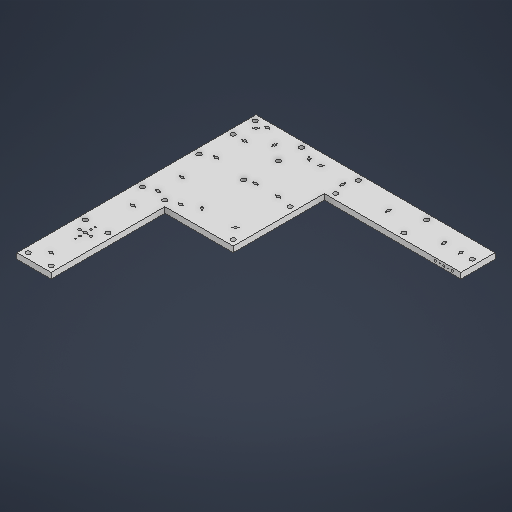
# Autodesk Inventor part: Baseplate Illum V3 L
Saved by Autodesk Inventor 2026 (Build 300175000, 175)
## iProperties
Created: 2026-02-09
Part Number: Baseplate Illum V3 L
Material: Generic
Document SubType Name: Modeling
Designer: FiolkaLab
Density: 1 g/cm^3
Appearance: Default
Author: FiolkaLab
Autodesk Inventor part; units mm, degrees
ref_plane "YZ Plane" through (0, 0, 0) normal (1, 0, 0) x (0, 1, 0)
ref_plane "XZ Plane" through (0, 0, 0) normal (0, 1, 0) x (-1, 0, 0)
ref_plane "XY Plane" through (0, 0, 0) normal (0, 0, 1) x (1, 0, 0)
sketch "Sketch1" plane through (0, 0, 0) normal (0, 1, 0) x (-1, 0, 0)
  line L0 (38.1, 0) -> (-38.1, 0)
  line L1 (-38.1, 0) -> (-38.1, 457.2)
  line L2 (-38.1, 457.2) -> (38.1, 457.2)
  line L3 (38.1, 457.2) -> (38.1, 0)
  point P0 (0, 0)
  dimension "d0" = 76.2
  dimension "d1" = 38.1
  dimension "d2" = 457.2
  constraints: 8 end point, 2 parallel, 1 horizontal, 1 perpendicular
  measures "d0" distance of L1.end L2.end
  measures "d1" distance of L0.start point (0, 0)
  measures "d2" distance of L2.end L0.start
extrude "Extrusion1" add sketch "Sketch1" along normal blind 12.7
sketch "Sketch2" plane through (0, 0, 0) normal (0, -1, 0) x (1, 0, 0)
  line L0 (38.1, 457.2) -> (38.1, 0) projected
  line L1 (-38.1, 457.2) -> (38.1, 457.2) projected
  point P0 (0, 0)
  point P1 (0, 419.1)
  dimension "d12" = 38.1
  dimension "d13" = 38.1
  measures "d12" distance from line of L0 point (0, 419.1)
  measures "d13" distance from line of L1 point (0, 419.1)
hole "Hole1" at (0, 0, 419.1) direction (0, 1, 0) diameter 6.35 end through all counterbore diameter 10.16 counterbore depth 7.62
sketch "Sketch3" plane through (0, 12.7, 0) normal (0, 1, 0) x (1, 0, 0)
  circle A0 centre (-5.004, -419.1) radius 1.0125
  circle A1 centre (5.004, -419.1) radius 1.0125
  circle A2 centre (0, -419.1) radius 3.175 projected
  point P0 (0, 0)
  dimension "d14" = 2.025
  dimension "d15" = 2.025
  dimension "d16" = 5.004
  dimension "d17" = 5.004
  constraints: 2 centre point
  measures "d14" diameter of A0
  measures "d15" diameter of A1
  measures "d16" distance of A2.centre A0.centre
  measures "d17" distance of A2.centre A1.centre
extrude "Extrusion2" cut sketch "Sketch3" against normal blind 4.445 contours A0 | A1
pattern_linear "Rectangular Pattern1" count 2 spacing 76.744 along (0, 0, -1) of "Hole1", "Extrusion2"
pattern_linear "Rectangular Pattern2" count 2 spacing 182.468 along (0, 0, -1) of "Hole1", "Extrusion2"
pattern_linear "Rectangular Pattern3" count 2 spacing 238.5038 along (0, 0, -1) of "Hole1", "Extrusion2"
sketch "Sketch5" plane through (0, 12.7, 0) normal (0, 1, 0) x (1, 0, 0)
  line L0 (38.1, 0) -> (-38.1, 0) projected
  line L1 (-38.1, 0) -> (495.3, 0)
  line L2 (495.3, 0) -> (495.3, 76.2)
  line L3 (495.3, 76.2) -> (-38.1, 76.2)
  line L4 (-38.1, 76.2) -> (-38.1, 0)
  point P0 (0, 0)
  point P1 (38.1, 0)
  dimension "d31" = 76.2
  dimension "d32" = 533.4
  constraints: 8 end point, 2 parallel, 1 horizontal, 1 perpendicular
  measures "d31" distance of L3.end L0.end
  measures "d32" distance of L2.end L3.end
extrude "Extrusion3" add sketch "Sketch5" against normal blind 12.7
sketch "Sketch6" plane through (0, 0, 0) normal (0, -1, 0) x (1, 0, 0)
  line L0 (-38.1, 457.2) -> (-38.1, -76.2) projected
  line L1 (-38.1, -76.2) -> (495.3, -76.2) projected
  point P0 (0, 0)
  point P1 (-12.0376, -50.1336)
  dimension "d42" = 26.0624
  dimension "d43" = 26.0664
  measures "d42" distance from line of L0 point (-12.038, -50.134)
  measures "d43" distance from line of L1 point (-12.038, -50.134)
hole "Hole2" at (-12.0376, 0, -50.1336) direction (0, 1, 0) diameter 6.35 end through all counterbore diameter 10.16 counterbore depth 7.62
sketch "Sketch11" plane through (0, 12.7, 0) normal (0, 1, 0) x (1, 0, 0)
  circle A0 centre (-17.0416, 46.9586) radius 1.0125
  circle A1 centre (-7.0336, 53.3086) radius 1.0125
  circle A2 centre (-12.0376, 50.1336) radius 3.175 projected
  circle A3 centre (-15.576, 46.5952) radius 1.0125
  circle A4 centre (-8.4992, 53.672) radius 1.0125
  point P0 (0, 0)
  dimension "d67" = 2.025
  dimension "d68" = 2.025
  dimension "d69" = 5.004
  dimension "d70" = 3.175
  dimension "d71" = 5.004
  dimension "d72" = 3.175
  dimension "d404" = 2.025
  dimension "d405" = 2.025
  dimension "d406" = 5.004
  dimension "d407" = 5.004
  constraints: 4 centre point
  measures "d67" diameter of A0
  measures "d68" diameter of A1
  measures "d69" horizontal distance of A2.centre A0.centre
  measures "d70" vertical distance of A2.centre A0.centre
  measures "d71" horizontal distance of A2.centre A1.centre
  measures "d72" vertical distance of A2.centre A1.centre
  measures "d404" diameter of A3
  measures "d405" diameter of A4
  measures "d406" distance of A2.centre A3.centre
  measures "d407" distance of A2.centre A4.centre
extrude "Extrusion6" [suppressed]
sketch "Sketch12" plane through (38.1, 0, 457.2) normal (1, 0, 0) x (0, 0, -1)
  line L0 (457.2, 0) -> (457.2, 12.7) projected
  line L1 (0, 0) -> (457.2, 0) projected
  line L2 (457.2, 12.7) -> (254, 12.7)
  line L3 (254, 12.7) -> (254, 0)
  line L4 (254, 0) -> (457.2, 0)
  line L5 (457.2, 0) -> (457.2, 12.7)
  dimension "d77" = 203.2
  constraints: 8 end point, 2 parallel, 1 horizontal, 1 perpendicular, 1 point on line
  measures "d77" distance of L4.end L3.end
extrude "Extrusion7" add sketch "Sketch12" along normal blind 152.4
sketch "Sketch13" plane through (0, 0, 0) normal (0, -1, 0) x (1, 0, 0)
  circle A0 centre (0, 180.5962) radius 5.08 projected
  line L0 (38.1, 203.2) -> (190.5, 203.2) projected
  point P0 (0, 0)
  point P1 (50.8, 180.7682)
  dimension "d87" = 50.8
  dimension "d318" = 0.172
  measures "d87" horizontal distance of A0.centre point (50.8, 180.768)
  measures "d318" vertical distance of point (50.8, 180.768) A0.centre
hole "Hole4" at (50.8, 0, 180.7682) direction (0, 1, 0) diameter 6.35 end through all counterbore diameter 10.16 counterbore depth 7.62
sketch "Sketch14" plane through (0, 12.7, 0) normal (0, 1, 0) x (1, 0, 0)
  circle A0 centre (45.796, -180.7682) radius 1.0125
  circle A1 centre (55.804, -180.7682) radius 1.0125
  circle A2 centre (50.8, -180.7682) radius 3.175 projected
  point P0 (0, 0)
  dimension "d88" = 2.025
  dimension "d89" = 2.025
  dimension "d90" = 5.004
  dimension "d91" = 5.004
  constraints: 2 centre point
  measures "d88" diameter of A0
  measures "d89" diameter of A1
  measures "d90" distance of A2.centre A0.centre
  measures "d91" distance of A2.centre A1.centre
extrude "Extrusion8" cut sketch "Sketch14" against normal blind 4.445 contours A0 | A1
sketch "Sketch15" plane through (0, 0, 0) normal (0, -1, 0) x (1, 0, 0)
  line L0 (495.3, 0) -> (190.5, 0) projected
  line L1 (-38.1, -76.2) -> (-38.1, 457.2) projected
  point P0 (0, 0)
  point P1 (40.935, -38.1)
  dimension "d101" = 38.1
  dimension "d117" = 79.035
  measures "d101" distance from line of L0 point (40.935, -38.1)
  measures "d117" distance from line of L1 point (40.935, -38.1)
hole "Hole5" at (40.935, 0, -38.1) direction (0, 1, 0) diameter 6.35 end through all counterbore diameter 10.16 counterbore depth 7.62
sketch "Sketch16" plane through (0, 12.7, 0) normal (0, 1, 0) x (1, 0, 0)
  circle A0 centre (40.935, 33.096) radius 1.0125
  circle A1 centre (40.935, 43.104) radius 1.0125
  circle A2 centre (40.935, 38.1) radius 3.175 projected
  point P0 (0, 0)
  dimension "d102" = 2.025
  dimension "d103" = 2.025
  dimension "d104" = 5.004
  dimension "d105" = 5.004
  constraints: 2 centre point
  measures "d102" diameter of A0
  measures "d103" diameter of A1
  measures "d104" distance of A2.centre A1.centre
  measures "d105" distance of A2.centre A0.centre
extrude "Extrusion9" cut sketch "Sketch16" against normal blind 4.445 contours A0 | A1
pattern_linear "Rectangular Pattern4" count 2 spacing 152.534 along (1, 0, 0) of "Hole5", "Extrusion9"
pattern_linear "Rectangular Pattern5" count 2 spacing 378.628 along (1, 0, 0) of "Hole5", "Extrusion9"
pattern_linear "Rectangular Pattern6" count 2 spacing 416.2604 along (1, 0, 0) of "Hole5", "Extrusion9"
sketch "Sketch17" plane through (495.3, 0, 0) normal (0, 0, 1) x (1, 0, 0)
  line L0 (0, 0) -> (-304.8, 0) projected
  line L1 (0, 12.7) -> (0, 0) projected
  point P0 (-495.3, 0)
  point P1 (-38.1, 6.35)
  dimension "d133" = 6.35
  dimension "d134" = 38.1
  measures "d133" distance from line of L0 point (-38.1, 6.35)
  measures "d134" distance from line of L1 point (-38.1, 6.35)
hole "Hole6" at (457.2, 6.35, 0) direction (0, 0, -1) diameter 4.9784 depth 12.7 thread size "1/4-20 UNC" class "2B" standard "ANSI Unified Screw Threads"
pattern_linear "Rectangular Pattern9" count 2 spacing 19.05 along (1, 0, 0) count 2 spacing 19.05 along (-1, 0, 0) of "Hole6"
sketch "Sketch18" plane through (495.3, 0, 0) normal (0, 0, 1) x (1, 0, 0)
  circle A0 centre (-47.625, 6.35) radius 1.0125
  circle A1 centre (-28.575, 6.35) radius 1.0125
  circle A2 centre (-38.1, 6.35) radius 2.4892 projected
  point P0 (-495.3, 0)
  dimension "d141" = 2.025
  dimension "d142" = 2.025
  dimension "d143" = 9.525
  dimension "d144" = 9.525
  constraints: 2 centre point
  measures "d141" diameter of A0
  measures "d142" diameter of A1
  measures "d143" distance of A2.centre A0.centre
  measures "d144" distance of A2.centre A1.centre
extrude "Extrusion10" cut sketch "Sketch18" against normal blind 3 contours A0 | A1
pattern_linear "Rectangular Pattern10" count 2 spacing 144.7 along (1, 0, 0) of "Hole2"
sketch "Sketch19" plane through (0, 0, 0) normal (0, -1, 0) x (1, 0, 0)
  line L0 (-38.1, 457.2) -> (-38.1, -76.2) projected
  line L1 (38.1, 203.2) -> (190.5, 203.2) projected
  circle A0 centre (50.8, 180.7682) radius 3.175 projected
  point P0 (0, 0)
  point P1 (82.55, 164.7072)
  dimension "d154" = 120.65
  dimension "d213" = 16.061
  measures "d154" distance from line of L0 point (82.55, 164.707)
  measures "d213" vertical distance of A0.centre point (82.55, 164.707)
hole "Hole7" at (82.55, 0, 164.7072) direction (0, 1, 0) diameter 6.35 end through all counterbore diameter 10.16 counterbore depth 7.62
sketch "Sketch22" plane through (0, 12.7, 0) normal (0, 1, 0) x (1, 0, 0)
  circle A0 centre (77.546, -161.5322) radius 1.0125
  circle A1 centre (87.554, -167.8822) radius 1.0125
  circle A2 centre (82.55, -164.7072) radius 3.175 projected
  circle A3 centre (79.0116, -161.1688) radius 1.0125
  circle A4 centre (86.0884, -168.2456) radius 1.0125
  point P0 (0, 0)
  dimension "d169" = 2.025
  dimension "d170" = 2.025
  dimension "d171" = 3.175
  dimension "d172" = 5.004
  dimension "d173" = 5.004
  dimension "d174" = 3.175
  dimension "d414" = 2.025
  dimension "d415" = 2.025
  dimension "d416" = 5.004
  dimension "d417" = 5.004
  constraints: 4 centre point
  measures "d169" diameter of A0
  measures "d170" diameter of A1
  measures "d171" vertical distance of A2.centre A0.centre
  measures "d172" horizontal distance of A2.centre A0.centre
  measures "d173" horizontal distance of A2.centre A1.centre
  measures "d174" vertical distance of A2.centre A1.centre
  measures "d414" diameter of A3
  measures "d415" diameter of A4
  measures "d416" distance of A2.centre A4.centre
  measures "d417" distance of A2.centre A3.centre
extrude "Extrusion11" [suppressed]
sketch "Sketch23" plane through (0, 0, 0) normal (0, -1, 0) x (1, 0, 0)
  line L0 (495.3, -76.2) -> (-38.1, -76.2) projected
  line L1 (-38.1, -76.2) -> (-38.1, 457.2) projected
  point P0 (0, 0)
  point P1 (106.6172, -50.1336)
  dimension "d191" = 26.0664
  dimension "d194" = 144.7172
  measures "d191" distance from line of L0 point (106.617, -50.134)
  measures "d194" distance from line of L1 point (106.617, -50.134)
hole "Hole8" at (106.6172, 0, -50.1336) direction (0, 1, 0) diameter 6.35 end through all counterbore diameter 10.16 counterbore depth 7.62
sketch "Sketch24" plane through (0, 12.7, 0) normal (0, 1, 0) x (1, 0, 0)
  circle A0 centre (101.6132, 53.3086) radius 1.0125
  circle A1 centre (111.6212, 46.9586) radius 1.0125
  circle A2 centre (106.6172, 50.1336) radius 3.175 projected
  circle A3 centre (103.0788, 53.672) radius 1.0125
  circle A4 centre (110.1556, 46.5952) radius 1.0125
  point P0 (0, 0)
  dimension "d185" = 2.025
  dimension "d186" = 2.025
  dimension "d187" = 5.004
  dimension "d188" = 5.004
  dimension "d189" = 3.175
  dimension "d190" = 3.175
  dimension "d408" = 2.025
  dimension "d409" = 2.025
  dimension "d412" = 5.004
  dimension "d413" = 5.004
  constraints: 4 centre point
  measures "d185" diameter of A0
  measures "d186" diameter of A1
  measures "d187" horizontal distance of A2.centre A0.centre
  measures "d188" horizontal distance of A2.centre A1.centre
  measures "d189" vertical distance of A2.centre A0.centre
  measures "d190" vertical distance of A2.centre A1.centre
  measures "d408" diameter of A3
  measures "d409" diameter of A4
  measures "d412" distance of A2.centre A3.centre
  measures "d413" distance of A4.centre A2.centre
extrude "Extrusion12" [suppressed]
sketch "Sketch25" plane through (0, 0, 0) normal (0, -1, 0) x (1, 0, 0)
  line L0 (38.1, 203.2) -> (190.5, 203.2) projected
  line L1 (-38.1, -76.2) -> (-38.1, 457.2) projected
  circle A0 centre (82.55, 164.7072) radius 3.175 projected
  point P0 (0, 0)
  point P1 (156.7298, 164.7072)
  dimension "d212" = 74.1798
  dimension "d214" = 0
  measures "d212" distance of A0.centre point (156.73, 164.707)
  measures "d214" vertical distance of A0.centre point (156.73, 164.707)
hole "Hole9" at (156.7298, 0, 164.7072) direction (0, 1, 0) diameter 6.35 end through all counterbore diameter 10.16 counterbore depth 7.62
sketch "Sketch26" plane through (0, 12.7, 0) normal (0, 1, 0) x (1, 0, 0)
  circle A0 centre (151.7258, -167.8822) radius 1.0125
  circle A1 centre (161.7338, -161.5322) radius 1.0125
  circle A2 centre (156.7298, -164.7072) radius 3.175 projected
  circle A3 centre (160.2682, -161.1688) radius 1.0125
  circle A4 centre (153.1914, -168.2456) radius 1.0125
  point P0 (0, 0)
  dimension "d204" = 2.025
  dimension "d205" = 2.025
  dimension "d206" = 3.175
  dimension "d207" = 5.004
  dimension "d208" = 3.175
  dimension "d209" = 5.004
  dimension "d418" = 2.025
  dimension "d419" = 2.025
  dimension "d420" = 5.004
  dimension "d421" = 5.004
  constraints: 4 centre point
  measures "d204" diameter of A0
  measures "d205" diameter of A1
  measures "d206" vertical distance of A2.centre A1.centre
  measures "d207" horizontal distance of A2.centre A0.centre
  measures "d208" vertical distance of A2.centre A0.centre
  measures "d209" horizontal distance of A2.centre A1.centre
  measures "d418" diameter of A3
  measures "d419" diameter of A4
  measures "d420" distance of A2.centre A4.centre
  measures "d421" distance of A2.centre A3.centre
extrude "Extrusion13" [suppressed]
sketch "Sketch30" plane through (0, 12.7, 0) normal (0, 1, 0) x (1, 0, 0)
  circle A0 centre (0, -342.356) radius 3.175 projected
  point P0 (0, 0)
  point P1 (0, -354.856)
  point P2 (0, -329.856)
  dimension "d326" = 12.5
  dimension "d327" = 12.5
  dimension "d330" = 0
  dimension "d333" = 0
  measures "d326" distance of A0.centre point (0, -354.856)
  measures "d327" distance of A0.centre point (0, -329.856)
  measures "d330" horizontal distance of point (0, -354.856) A0.centre
  measures "d333" horizontal distance of A0.centre point (0, -329.856)
hole "Hole13" at (0, 12.7, 354.856) at (0, 12.7, 329.856) direction (0, -1, 0) diameter 4.9784 end through all thread size "1/4-20 UNC" class "2B" standard "ANSI Unified Screw Threads"
sketch "Sketch32" plane through (0, 0, 0) normal (0, -1, 0) x (1, 0, 0)
  circle A0 centre (0, 342.356) radius 5.08 projected
  point P0 (0, 0)
  point P1 (-12.5, 342.356)
  point P2 (12.5, 342.356)
  dimension "d352" = 0
  dimension "d353" = 0
  dimension "d354" = 12.5
  dimension "d355" = 12.5
  measures "d352" vertical distance of A0.centre point (12.5, 342.356)
  measures "d353" vertical distance of A0.centre point (-12.5, 342.356)
  measures "d354" distance of A0.centre point (-12.5, 342.356)
  measures "d355" distance of A0.centre point (12.5, 342.356)
hole "Hole15" at (-12.5, 0, 342.356) at (12.5, 0, 342.356) direction (0, 1, 0) diameter 6.35 end through all counterbore diameter 10.16 counterbore depth 7.62
sketch "Sketch33" plane through (0, 12.7, 0) normal (0, 1, 0) x (1, 0, 0)
  circle A0 centre (0, -320.352) radius 1.5125
  circle A1 centre (0, -364.36) radius 1.5125
  circle A2 centre (0, -342.356) radius 3.175 projected
  point P0 (0, 0)
  dimension "d356" = 3.025
  dimension "d357" = 3.025
  dimension "d358" = 22.004
  dimension "d359" = 22.004
  constraints: 2 centre point
  measures "d356" diameter of A0
  measures "d357" diameter of A1
  measures "d358" distance of A2.centre A0.centre
  measures "d359" distance of A2.centre A1.centre
extrude "Extrusion14" cut sketch "Sketch33" against normal blind 4.5 contours A0 | A1
sketch "Sketch34" plane through (0, 12.7, 0) normal (0, 1, 0) x (1, 0, 0)
  line L0 (-38.1, 76.2) -> (-38.1, -457.2) projected
  line L1 (-38.1, -457.2) -> (38.1, -457.2) projected
  line L2 (38.1, -457.2) -> (38.1, -203.2) projected
  line L3 (190.5, 0) -> (190.5, -203.2) projected
  line L4 (495.3, 0) -> (495.3, 76.2) projected
  line L5 (190.5, 0) -> (495.3, 0) projected
  line L6 (495.3, 76.2) -> (-38.1, 76.2) projected
  point P0 (0, 0)
  point P1 (-25.4, -444.5)
  point P2 (25.4, -444.5)
  point P3 (-25.4, -317.5)
  point P4 (25.4, -317.5)
  point P5 (25.4, -190.5)
  point P6 (-25.4, -190.5)
  point P7 (177.8, -190.5)
  point P8 (-25.4, -63.5)
  point P9 (74.2174, -63.5)
  point P10 (177.8, -63.5)
  point P11 (482.6, 38.1)
  point P12 (355.6, 12.7)
  point P13 (355.6, 63.5)
  point P14 (203.2, 12.7)
  point P15 (203.2, 63.5)
  point P16 (76.2, 11.2809)
  point P17 (76.2, 63.5)
  point P18 (-27.1997, 63.5)
  point P19 (-25.4, 12.7)
  dimension "d369" = 12.7
  dimension "d370" = 12.7
  dimension "d371" = 12.7
  dimension "d372" = 12.7
  dimension "d373" = 12.7
  dimension "d374" = 127
  dimension "d375" = 12.7
  dimension "d376" = 127
  dimension "d377" = 127
  dimension "d378" = 12.7
  dimension "d379" = 12.7
  dimension "d380" = 127
  dimension "d381" = 127
  dimension "d382" = 127
  dimension "d383" = 12.7
  dimension "d384" = 127
  dimension "d385" = 152.4
  dimension "d386" = 127
  dimension "d387" = 12.7
  dimension "d388" = 127
  dimension "d389" = 12.7
  dimension "d390" = 38.1
  dimension "d391" = 127
  dimension "d392" = 127
  dimension "d393" = 12.7
  dimension "d394" = 12.7
  dimension "d395" = 152.4
  dimension "d396" = 152.4
  dimension "d397" = 12.7
  dimension "d398" = 12.7
  dimension "d399" = 127
  dimension "d400" = 127
  dimension "d401" = 12.7
  dimension "d402" = 76.2
  dimension "d403" = 12.7
  measures "d369" distance from line of L0 point (-25.4, -444.5)
  measures "d370" distance from line of L1 point (-25.4, -444.5)
  measures "d371" distance from line of L1 point (25.4, -444.5)
  measures "d372" distance from line of L2 point (25.4, -444.5)
  measures "d373" distance from line of L2 point (25.4, -317.5)
  measures "d374" distance of point (25.4, -444.5) point (25.4, -317.5)
  measures "d375" distance from line of L0 point (-25.4, -317.5)
  measures "d376" distance of point (-25.4, -444.5) point (-25.4, -317.5)
  measures "d377" distance of point (25.4, -317.5) point (25.4, -190.5)
  measures "d378" distance from line of L2 point (25.4, -190.5)
  measures "d379" distance from line of L0 point (-25.4, -190.5)
  measures "d380" distance of point (-25.4, -317.5) point (-25.4, -190.5)
  measures "d381" distance of point (-25.4, -190.5) point (-25.4, -63.5)
  measures "d382" vertical distance of point (25.4, -190.5) point (74.217, -63.5)
  measures "d383" distance from line of L0 point (-25.4, -63.5)
  measures "d384" vertical distance of point (177.8, -190.5) point (25.4, -317.5)
  measures "d385" distance of point (177.8, -190.5) point (25.4, -190.5)
  measures "d386" distance of point (177.8, -63.5) point (177.8, -190.5)
  measures "d387" distance from line of L3 point (177.8, -63.5)
  measures "d388" vertical distance of point (-27.2, 63.5) point (-25.4, -63.5)
  measures "d389" distance from line of L4 point (482.6, 38.1)
  measures "d390" distance from line of L5 point (482.6, 38.1)
  measures "d391" horizontal distance of point (482.6, 38.1) point (355.6, 12.7)
  measures "d392" horizontal distance of point (482.6, 38.1) point (355.6, 63.5)
  measures "d393" distance from line of L6 point (355.6, 63.5)
  measures "d394" distance from line of L5 point (355.6, 12.7)
  measures "d395" distance of point (355.6, 12.7) point (203.2, 12.7)
  measures "d396" distance of point (355.6, 63.5) point (203.2, 63.5)
  measures "d397" distance from line of L6 point (203.2, 63.5)
  measures "d398" distance from line of L5 point (203.2, 12.7)
  measures "d399" horizontal distance of point (203.2, 12.7) point (76.2, 11.281)
  measures "d400" distance of point (203.2, 63.5) point (76.2, 63.5)
  measures "d401" distance from line of L6 point (76.2, 63.5)
  measures "d402" distance of point (-25.4, 12.7) point (-25.4, -63.5)
  measures "d403" distance from line of L0 point (-25.4, 12.7)
hole "Hole16" at (-25.4, 12.7, 444.5) at (25.4, 12.7, 444.5) at (-25.4, 12.7, 317.5) at (25.4, 12.7, 317.5) at (25.4, 12.7, 190.5) at (-25.4, 12.7, 190.5) at (177.8, 12.7, 190.5) at (-25.4, 12.7, 63.5) at (74.2174, 12.7, 63.5) at (177.8, 12.7, 63.5) at (482.6, 12.7, -38.1) at (355.6, 12.7, -12.7) at (355.6, 12.7, -63.5) at (203.2, 12.7, -12.7) at (203.2, 12.7, -63.5) at (76.2, 12.7, -11.2809) at (76.2, 12.7, -63.5) at (-27.1997, 12.7, -63.5) at (-25.4, 12.7, -12.7) direction (0, -1, 0) diameter 6.35 end through all counterbore diameter 10.16 counterbore depth 7.62
sketch "Sketch35" plane through (0, 12.7, 0) normal (0, 1, 0) x (1, 0, 0)
  circle A0 centre (-8.4992, 53.672) radius 1.0125
  circle A1 centre (-15.576, 46.5952) radius 1.0125
  circle A2 centre (103.0788, 53.672) radius 1.0125
  circle A3 centre (110.1556, 46.5952) radius 1.0125
  circle A4 centre (86.0884, -168.2456) radius 1.0125
  circle A5 centre (79.0116, -161.1688) radius 1.0125
  circle A6 centre (153.1914, -168.2456) radius 1.0125
  circle A7 centre (160.2682, -161.1688) radius 1.0125
  circle A8 centre (136.2008, 53.672) radius 1.0125
  circle A9 centre (129.124, 46.5952) radius 1.0125
  circle A10 centre (-12.0376, 50.1336) radius 3.175 projected
  circle A11 centre (106.6172, 50.1336) radius 3.175 projected
  circle A12 centre (82.55, -164.7072) radius 3.175 projected
  circle A13 centre (156.7298, -164.7072) radius 3.175 projected
  circle A14 centre (132.6624, 50.1336) radius 3.175 projected
  circle A15 centre (132.6624, 50.1336) radius 3.175
  point P0 (0, 0)
  dimension "d422" = 2.025
  dimension "d423" = 2.025
  dimension "d424" = 2.025
  dimension "d425" = 2.025
  dimension "d426" = 2.025
  dimension "d427" = 2.025
  dimension "d428" = 2.025
  dimension "d429" = 2.025
  dimension "d430" = 2.025
  dimension "d431" = 2.025
  dimension "d432" = 5.004
  dimension "d433" = 5.004
  dimension "d434" = 5.004
  dimension "d435" = 5.004
  dimension "d436" = 5.004
  dimension "d437" = 5.004
  dimension "d438" = 5.004
  dimension "d439" = 5.004
  dimension "d440" = 5.004
  dimension "d441" = 5.004
  constraints: 11 centre point, 1 coincident, 1 concentric
  measures "d422" diameter of A0
  measures "d423" diameter of A1
  measures "d424" diameter of A2
  measures "d425" diameter of A3
  measures "d426" diameter of A4
  measures "d427" diameter of A5
  measures "d428" diameter of A6
  measures "d429" diameter of A7
  measures "d430" diameter of A8
  measures "d431" diameter of A9
  measures "d432" distance of A10.centre A1.centre
  measures "d433" distance of A10.centre A0.centre
  measures "d434" distance of A11.centre A2.centre
  measures "d435" distance of A11.centre A3.centre
  measures "d436" distance of A12.centre A5.centre
  measures "d437" distance of A12.centre A4.centre
  measures "d438" distance of A13.centre A7.centre
  measures "d439" distance of A13.centre A6.centre
  measures "d440" distance of A14.centre A8.centre
  measures "d441" distance of A14.centre A9.centre
extrude "Extrusion15" cut sketch "Sketch35" against normal blind 4.445 contours A0 | A1 | A2 | A3 | A4 | A5 | A6 | A7 | A8 | A9
pattern_linear "Rectangular Pattern11" count 2 spacing 292.1 along (0, 0, -1) of "Hole1", "Extrusion2"
pattern_linear "Rectangular Pattern14" count 2 spacing 254 along (1, 0, 0) of "Hole5", "Extrusion9"
pattern_linear "Rectangular Pattern15" count 2 spacing 368.3 along (0, 0, -1) of "Hole1", "Extrusion2"
pattern_linear "Rectangular Pattern16" count 2 spacing 482.6 along (0, 0, -1) of "Hole1", "Extrusion2"
pattern_linear "Rectangular Pattern17" count 2 spacing 431.8 along (0, 0, -1) of "Extrusion2", "Hole1"
sketch "Sketch36" plane through (0, 0, 0) normal (0, -1, 0) x (1, 0, 0)
  circle A0 centre (106.6172, -50.1336) radius 3.175 projected
  circle A1 centre (82.55, 164.7072) radius 5.08 projected
  point P0 (0, 0)
  point P1 (94.5835, 57.2869)
  dimension "d472" = 107.4205
  dimension "d473" = 12.0335
  measures "d472" vertical distance of A0.centre point (94.584, 57.287)
  measures "d473" horizontal distance of A1.centre point (94.584, 57.287)
hole "Hole17" at (94.5835, 0, 57.2869) direction (0, 1, 0) diameter 6.35 end through all counterbore diameter 10.16 counterbore depth 7.62
sketch "Sketch37" plane through (0, 12.7, 0) normal (0, 1, 0) x (1, 0, 0)
  circle A0 centre (99.5875, -57.2869) radius 1.0125
  circle A1 centre (89.5795, -57.2869) radius 1.0125
  circle A2 centre (94.5835, -57.2869) radius 3.175 projected
  point P0 (0, 0)
  dimension "d474" = 2.025
  dimension "d475" = 2.025
  dimension "d476" = 5.004
  dimension "d477" = 5.004
  constraints: 2 centre point
  measures "d474" diameter of A0
  measures "d475" diameter of A1
  measures "d476" distance of A2.centre A1.centre
  measures "d477" distance of A2.centre A0.centre
extrude "Extrusion16" cut sketch "Sketch37" against normal blind 4.445 contours A0 | A1
pattern_linear "Rectangular Pattern18" count 2 spacing 50.112 along (1, 0, 0) of "Hole17", "Extrusion16"
body "Solid1"
